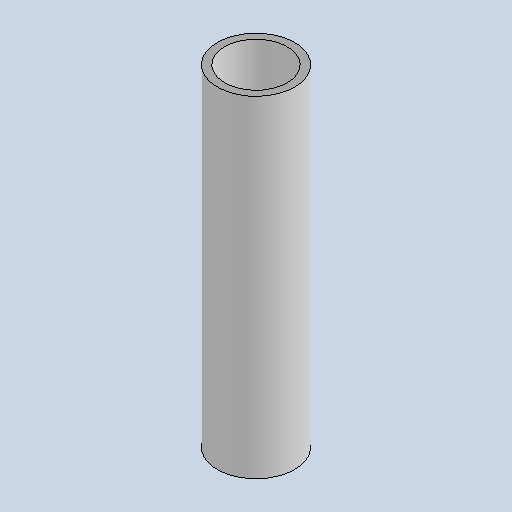
# Autodesk Inventor part: TZS 1756 FDS 940 way tube 6
Saved by Autodesk Inventor 2025.1 (Build 291241020, 241B)
## iProperties
Created: 2025-06-24
Part Number: TZS 1756 FDS 940 way tube 6
Material: Stainless Steel
Document SubType Name: Modeling
Designer: user
Mass: 1762.25 g
Surface Area: 2283.33 cm^2
Volume: 220.281 cm^3
Density: 8 g/cm^3
Sheet Metal Width: 0.000 mm
Sheet Metal Length: 0.000 mm
Sheet Metal Area: 0.000 mm^2
Appearance: Default
Sheet Metal Rule: AISI304 2mm Die16
Author: user
Autodesk Inventor part; units mm, degrees
ref_plane "YZ Plane" through (0, 0, 0) normal (1, 0, 0) x (0, 1, 0)
ref_plane "XZ Plane" through (0, 0, 0) normal (0, 1, 0) x (-1, 0, 0)
ref_plane "XY Plane" through (0, 0, 0) normal (0, 0, 1) x (1, 0, 0)
sketch "Sketch11" plane through (0, 0, 0) normal (0, 0, 1) x (1, 0, 0)
  circle A0 centre (0, 0) radius 10.5
  circle A1 centre (0, 0) radius 8.5
  dimension "d187" = 21
  dimension "d188" = 2
  constraints: 2 centre point, 1 coincident
  measures "d187" diameter of A0
  measures "d188" radial gap between concentric circles of A0 A1
extrude "Extrusion5" add sketch "Sketch11" against normal blind 90
body "Solid5"
